Autodesk Fusion 360 part; units mm, degrees
(part 3 of 6)
  spline S37 degree 5 poles (53.0142, 47.6687) (53.0234, 47.6622) (53.0419, 47.6493) (53.0695, 47.6299) (53.1065, 47.6042) (53.1527, 47.5723) (53.1991, 47.5406) (53.2455, 47.5092) (53.292, 47.478) (53.3386, 47.4471) (53.3852, 47.4164) (53.4319, 47.3859) (53.4787, 47.3557) (53.5256, 47.3258) (53.5726, 47.2961) (53.6196, 47.2667) (53.6667, 47.2375) (53.7139, 47.2086) (53.7612, 47.1799) (53.8085, 47.1515) (53.8559, 47.1233) (53.9034, 47.0955) (53.951, 47.0679) (53.9986, 47.0405) (54.0463, 47.0135) (54.0941, 46.9867) (54.142, 46.9602) (54.1899, 46.9339) (54.2379, 46.908) (54.286, 46.8823) (54.3341, 46.8569) (54.3823, 46.8318) (54.4306, 46.807) (54.4789, 46.7825) (54.5273, 46.7583) (54.5758, 46.7344) (54.6244, 46.7108) (54.673, 46.6875) (54.7217, 46.6646) (54.7704, 46.6419) (54.8193, 46.6196) (54.8682, 46.5976) (54.9171, 46.5759) (54.9662, 46.5546) (55.0152, 46.5336) (55.0644, 46.5129) (55.1136, 46.4926) (55.1629, 46.4726) (55.2123, 46.453) (55.2617, 46.4338) (55.3112, 46.4149) (55.3607, 46.3965) (55.4103, 46.3784) (55.46, 46.3608) (55.5098, 46.3436) (55.5596, 46.3268) (55.6095, 46.3104) (55.6594, 46.2943) (55.7094, 46.2787) (55.7594, 46.2635) (55.8095, 46.2488) (55.8597, 46.2348) (55.91, 46.2215) (55.9604, 46.2089) (56.0108, 46.1968) (56.0613, 46.1852) (56.1118, 46.1739) (56.1624, 46.163) (56.213, 46.1525) (56.2636, 46.143) (56.3144, 46.1348) (56.3552, 46.1299) (56.3859, 46.1272) (56.4064, 46.126) (56.4167, 46.1255) knots -1 -1 -1 -1 -1 -1 -0.98571429 -0.97142857 -0.95714286 -0.94285714 -0.92857143 -0.91428571 -0.9 -0.88571429 -0.87142857 -0.85714286 -0.84285714 -0.82857143 -0.81428571 -0.8 -0.78571429 -0.77142857 -0.75714286 -0.74285714 -0.72857143 -0.71428571 -0.7 -0.68571429 -0.67142857 -0.65714286 -0.64285714 -0.62857143 -0.61428571 -0.6 -0.58571429 -0.57142857 -0.55714286 -0.54285714 -0.52857143 -0.51428571 -0.5 -0.48571429 -0.47142857 -0.45714286 -0.44285714 -0.42857143 -0.41428571 -0.4 -0.38571429 -0.37142857 -0.35714286 -0.34285714 -0.32857143 -0.31428571 -0.3 -0.28571429 -0.27142857 -0.25714286 -0.24285714 -0.22857143 -0.21428571 -0.2 -0.18571429 -0.17142857 -0.15714286 -0.14285714 -0.12857143 -0.11428571 -0.1 -0.08571429 -0.07142857 -0.05714286 -0.04285714 -0.02857143 -0.01428571 0 0 0 0 0 0
  line L37 (56.4167, 46.1255) -> (56.9142, 46.1012)
  arc A75 (57.3897, 45.5888) -> (56.9142, 46.1012) centre (56.8899, 45.6018) ccw
  arc A76 (57.3897, 45.5888) -> (57.3897, 44.4112) centre (79.882, 45) ccw
  arc A77 (56.9142, 43.8988) -> (57.3897, 44.4112) centre (56.8899, 44.3982) ccw
  line L38 (56.9142, 43.8988) -> (56.4167, 43.8745)
  spline S38 degree 5 poles (56.4167, 43.8745) (56.4064, 43.874) (56.3859, 43.8728) (56.3552, 43.8701) (56.3144, 43.8652) (56.2636, 43.857) (56.213, 43.8475) (56.1624, 43.837) (56.1118, 43.8261) (56.0613, 43.8148) (56.0108, 43.8032) (55.9604, 43.7911) (55.91, 43.7785) (55.8597, 43.7652) (55.8095, 43.7512) (55.7594, 43.7365) (55.7094, 43.7213) (55.6594, 43.7057) (55.6095, 43.6896) (55.5596, 43.6732) (55.5098, 43.6564) (55.46, 43.6392) (55.4103, 43.6216) (55.3607, 43.6035) (55.3112, 43.5851) (55.2617, 43.5662) (55.2123, 43.547) (55.1629, 43.5274) (55.1136, 43.5074) (55.0644, 43.4871) (55.0152, 43.4664) (54.9662, 43.4454) (54.9171, 43.4241) (54.8682, 43.4024) (54.8193, 43.3804) (54.7704, 43.3581) (54.7217, 43.3354) (54.673, 43.3125) (54.6244, 43.2892) (54.5758, 43.2656) (54.5273, 43.2417) (54.4789, 43.2175) (54.4306, 43.193) (54.3823, 43.1682) (54.3341, 43.1431) (54.286, 43.1177) (54.2379, 43.092) (54.1899, 43.0661) (54.142, 43.0398) (54.0941, 43.0133) (54.0463, 42.9865) (53.9986, 42.9595) (53.951, 42.9321) (53.9034, 42.9045) (53.8559, 42.8767) (53.8085, 42.8485) (53.7612, 42.8201) (53.7139, 42.7914) (53.6667, 42.7625) (53.6196, 42.7333) (53.5726, 42.7039) (53.5256, 42.6742) (53.4787, 42.6443) (53.4319, 42.6141) (53.3852, 42.5836) (53.3386, 42.5529) (53.292, 42.522) (53.2455, 42.4908) (53.1991, 42.4594) (53.1527, 42.4277) (53.1065, 42.3958) (53.0695, 42.3701) (53.0419, 42.3507) (53.0234, 42.3378) (53.0142, 42.3313) knots 0 0 0 0 0 0 0.01428571 0.02857143 0.04285714 0.05714286 0.07142857 0.08571429 0.1 0.11428571 0.12857143 0.14285714 0.15714286 0.17142857 0.18571429 0.2 0.21428571 0.22857143 0.24285714 0.25714286 0.27142857 0.28571429 0.3 0.31428571 0.32857143 0.34285714 0.35714286 0.37142857 0.38571429 0.4 0.41428571 0.42857143 0.44285714 0.45714286 0.47142857 0.48571429 0.5 0.51428571 0.52857143 0.54285714 0.55714286 0.57142857 0.58571429 0.6 0.61428571 0.62857143 0.64285714 0.65714286 0.67142857 0.68571429 0.7 0.71428571 0.72857143 0.74285714 0.75714286 0.77142857 0.78571429 0.8 0.81428571 0.82857143 0.84285714 0.85714286 0.87142857 0.88571429 0.9 0.91428571 0.92857143 0.94285714 0.95714286 0.97142857 0.98571429 1 1 1 1 1 1
  arc A78 (53.0142, 42.3313) -> (53.1946, 40.9031) centre (79.882, 45) ccw
  spline S39 degree 5 poles (53.1946, 40.9031) (53.2052, 40.8991) (53.2263, 40.8912) (53.2579, 40.8793) (53.3001, 40.8635) (53.3528, 40.8441) (53.4055, 40.825) (53.4583, 40.8061) (53.5111, 40.7875) (53.5639, 40.7691) (53.6167, 40.751) (53.6696, 40.7331) (53.7224, 40.7155) (53.7753, 40.6982) (53.8281, 40.6811) (53.881, 40.6643) (53.9339, 40.6477) (53.9868, 40.6314) (54.0397, 40.6154) (54.0926, 40.5997) (54.1455, 40.5842) (54.1985, 40.569) (54.2514, 40.5541) (54.3043, 40.5395) (54.3573, 40.5251) (54.4102, 40.5111) (54.4632, 40.4973) (54.5161, 40.4838) (54.569, 40.4706) (54.622, 40.4577) (54.6749, 40.4451) (54.7279, 40.4328) (54.7808, 40.4207) (54.8337, 40.409) (54.8866, 40.3976) (54.9395, 40.3865) (54.9924, 40.3758) (55.0453, 40.3653) (55.0982, 40.3552) (55.151, 40.3453) (55.2039, 40.3358) (55.2567, 40.3267) (55.3095, 40.3179) (55.3623, 40.3094) (55.4151, 40.3013) (55.4679, 40.2935) (55.5206, 40.2861) (55.5733, 40.279) (55.626, 40.2723) (55.6786, 40.2659) (55.7312, 40.2599) (55.7838, 40.2544) (55.8364, 40.2493) (55.8889, 40.2446) (55.9413, 40.2403) (55.9938, 40.2364) (56.0461, 40.2329) (56.0985, 40.2297) (56.1508, 40.227) (56.2031, 40.2247) (56.2552, 40.223) (56.3073, 40.2219) (56.3594, 40.2215) (56.4113, 40.2218) (56.4632, 40.2227) (56.5149, 40.224) (56.5667, 40.2256) (56.6183, 40.2276) (56.6699, 40.2301) (56.7214, 40.2334) (56.7726, 40.2381) (56.8133, 40.2435) (56.8437, 40.2486) (56.8639, 40.2525) (56.874, 40.2545) knots -1 -1 -1 -1 -1 -1 -0.98571429 -0.97142857 -0.95714286 -0.94285714 -0.92857143 -0.91428571 -0.9 -0.88571429 -0.87142857 -0.85714286 -0.84285714 -0.82857143 -0.81428571 -0.8 -0.78571429 -0.77142857 -0.75714286 -0.74285714 -0.72857143 -0.71428571 -0.7 -0.68571429 -0.67142857 -0.65714286 -0.64285714 -0.62857143 -0.61428571 -0.6 -0.58571429 -0.57142857 -0.55714286 -0.54285714 -0.52857143 -0.51428571 -0.5 -0.48571429 -0.47142857 -0.45714286 -0.44285714 -0.42857143 -0.41428571 -0.4 -0.38571429 -0.37142857 -0.35714286 -0.34285714 -0.32857143 -0.31428571 -0.3 -0.28571429 -0.27142857 -0.25714286 -0.24285714 -0.22857143 -0.21428571 -0.2 -0.18571429 -0.17142857 -0.15714286 -0.14285714 -0.12857143 -0.11428571 -0.1 -0.08571429 -0.07142857 -0.05714286 -0.04285714 -0.02857143 -0.01428571 0 0 0 0 0 0
  line L39 (56.874, 40.2545) -> (57.3619, 40.3548)
  arc A79 (57.9499, 39.9767) -> (57.3619, 40.3548) centre (57.4626, 39.865) ccw
  arc A80 (57.9499, 39.9767) -> (58.2428, 38.8361) centre (79.882, 45) ccw
  arc A81 (57.9097, 38.2215) -> (58.2428, 38.8361) centre (57.7619, 38.6992) ccw
  line L40 (57.9097, 38.2215) -> (57.4338, 38.0743)
  spline S40 degree 5 poles (57.4338, 38.0743) (57.424, 38.0712) (57.4044, 38.0649) (57.3753, 38.0547) (57.337, 38.0398) (57.2899, 38.0193) (57.2432, 37.9974) (57.1968, 37.9747) (57.1506, 37.9515) (57.1044, 37.9281) (57.0584, 37.9043) (57.0126, 37.88) (56.9669, 37.8553) (56.9215, 37.8299) (56.8764, 37.8038) (56.8315, 37.7772) (56.7868, 37.75) (56.7423, 37.7224) (56.6979, 37.6944) (56.6537, 37.6661) (56.6096, 37.6375) (56.5657, 37.6084) (56.522, 37.579) (56.4784, 37.5492) (56.435, 37.519) (56.3917, 37.4884) (56.3487, 37.4575) (56.3057, 37.4262) (56.263, 37.3946) (56.2203, 37.3627) (56.1779, 37.3305) (56.1355, 37.298) (56.0934, 37.2651) (56.0513, 37.2319) (56.0094, 37.1985) (55.9677, 37.1647) (55.9261, 37.1306) (55.8847, 37.0962) (55.8434, 37.0616) (55.8022, 37.0267) (55.7612, 36.9915) (55.7203, 36.956) (55.6796, 36.9202) (55.639, 36.8842) (55.5985, 36.8479) (55.5582, 36.8114) (55.518, 36.7745) (55.478, 36.7375) (55.4381, 36.7001) (55.3984, 36.6626) (55.3587, 36.6247) (55.3193, 36.5866) (55.2799, 36.5483) (55.2407, 36.5097) (55.2017, 36.4709) (55.1627, 36.4319) (55.1239, 36.3926) (55.0853, 36.3531) (55.0468, 36.3133) (55.0084, 36.2734) (54.9702, 36.2331) (54.9321, 36.1927) (54.8941, 36.152) (54.8563, 36.1112) (54.8186, 36.07) (54.781, 36.0287) (54.7436, 35.9872) (54.7063, 35.9454) (54.6692, 35.9034) (54.6322, 35.8613) (54.5953, 35.8189) (54.5659, 35.7848) (54.544, 35.7591) (54.5293, 35.7419) (54.522, 35.7334) knots 0 0 0 0 0 0 0.01428571 0.02857143 0.04285714 0.05714286 0.07142857 0.08571429 0.1 0.11428571 0.12857143 0.14285714 0.15714286 0.17142857 0.18571429 0.2 0.21428571 0.22857143 0.24285714 0.25714286 0.27142857 0.28571429 0.3 0.31428571 0.32857143 0.34285714 0.35714286 0.37142857 0.38571429 0.4 0.41428571 0.42857143 0.44285714 0.45714286 0.47142857 0.48571429 0.5 0.51428571 0.52857143 0.54285714 0.55714286 0.57142857 0.58571429 0.6 0.61428571 0.62857143 0.64285714 0.65714286 0.67142857 0.68571429 0.7 0.71428571 0.72857143 0.74285714 0.75714286 0.77142857 0.78571429 0.8 0.81428571 0.82857143 0.84285714 0.85714286 0.87142857 0.88571429 0.9 0.91428571 0.92857143 0.94285714 0.95714286 0.97142857 0.98571429 1 1 1 1 1 1
  arc A82 (54.522, 35.7334) -> (55.0519, 34.395) centre (79.882, 45) ccw
  spline S41 degree 5 poles (55.0519, 34.395) (55.0631, 34.3937) (55.0855, 34.3912) (55.1191, 34.3876) (55.1639, 34.3828) (55.2198, 34.3772) (55.2756, 34.3717) (55.3314, 34.3666) (55.3872, 34.3616) (55.4429, 34.357) (55.4986, 34.3526) (55.5542, 34.3484) (55.6098, 34.3445) (55.6653, 34.3408) (55.7207, 34.3374) (55.7761, 34.3343) (55.8315, 34.3314) (55.8868, 34.3288) (55.942, 34.3265) (55.9972, 34.3244) (56.0523, 34.3225) (56.1073, 34.321) (56.1623, 34.3197) (56.2172, 34.3187) (56.272, 34.318) (56.3268, 34.3175) (56.3815, 34.3173) (56.4362, 34.3174) (56.4907, 34.3178) (56.5452, 34.3185) (56.5996, 34.3194) (56.654, 34.3207) (56.7082, 34.3222) (56.7624, 34.324) (56.8165, 34.3261) (56.8705, 34.3285) (56.9244, 34.3313) (56.9782, 34.3343) (57.0319, 34.3376) (57.0856, 34.3412) (57.1391, 34.3452) (57.1926, 34.3494) (57.2459, 34.354) (57.2992, 34.359) (57.3523, 34.3642) (57.4053, 34.3698) (57.4582, 34.3757) (57.5111, 34.382) (57.5638, 34.3886) (57.6163, 34.3955) (57.6688, 34.4028) (57.7211, 34.4105) (57.7733, 34.4186) (57.8253, 34.4271) (57.8772, 34.436) (57.9289, 34.4453) (57.9805, 34.4549) (58.032, 34.4649) (58.0834, 34.4752) (58.1345, 34.486) (58.1855, 34.4974) (58.2362, 34.5093) (58.2867, 34.5218) (58.337, 34.535) (58.387, 34.5487) (58.4368, 34.5629) (58.4865, 34.5773) (58.5361, 34.5921) (58.5854, 34.6073) (58.6344, 34.6233) (58.6829, 34.6407) (58.721, 34.656) (58.7491, 34.6685) (58.7677, 34.6773) (58.777, 34.6818) knots -1 -1 -1 -1 -1 -1 -0.98571429 -0.97142857 -0.95714286 -0.94285714 -0.92857143 -0.91428571 -0.9 -0.88571429 -0.87142857 -0.85714286 -0.84285714 -0.82857143 -0.81428571 -0.8 -0.78571429 -0.77142857 -0.75714286 -0.74285714 -0.72857143 -0.71428571 -0.7 -0.68571429 -0.67142857 -0.65714286 -0.64285714 -0.62857143 -0.61428571 -0.6 -0.58571429 -0.57142857 -0.55714286 -0.54285714 -0.52857143 -0.51428571 -0.5 -0.48571429 -0.47142857 -0.45714286 -0.44285714 -0.42857143 -0.41428571 -0.4 -0.38571429 -0.37142857 -0.35714286 -0.34285714 -0.32857143 -0.31428571 -0.3 -0.28571429 -0.27142857 -0.25714286 -0.24285714 -0.22857143 -0.21428571 -0.2 -0.18571429 -0.17142857 -0.15714286 -0.14285714 -0.12857143 -0.11428571 -0.1 -0.08571429 -0.07142857 -0.05714286 -0.04285714 -0.02857143 -0.01428571 0 0 0 0 0 0
  line L41 (58.777, 34.6818) -> (59.2247, 34.9002)
  arc A83 (59.8882, 34.6802) -> (59.2247, 34.9002) centre (59.4439, 34.4509) ccw
  arc A84 (59.8882, 34.6802) -> (60.4555, 33.6483) centre (79.882, 45) ccw
  arc A85 (60.2857, 32.9702) -> (60.4555, 33.6483) centre (60.0238, 33.3961) ccw
  line L42 (60.2857, 32.9702) -> (59.8614, 32.7092)
  spline S42 degree 5 poles (59.8614, 32.7092) (59.8526, 32.7038) (59.8353, 32.6928) (59.8096, 32.6757) (59.7763, 32.6518) (59.7357, 32.6202) (59.6959, 32.5874) (59.6566, 32.5538) (59.6176, 32.5199) (59.5788, 32.4857) (59.5401, 32.4512) (59.5017, 32.4163) (59.4637, 32.381) (59.426, 32.3451) (59.3888, 32.3086) (59.3519, 32.2717) (59.3154, 32.2342) (59.2791, 32.1964) (59.2431, 32.1583) (59.2073, 32.1199) (59.1718, 32.0812) (59.1364, 32.0421) (59.1014, 32.0028) (59.0666, 31.9631) (59.0321, 31.923) (58.9978, 31.8826) (58.9638, 31.842) (58.93, 31.801) (58.8964, 31.7598) (58.863, 31.7182) (58.8299, 31.6765) (58.797, 31.6344) (58.7643, 31.5921) (58.7318, 31.5495) (58.6996, 31.5067) (58.6676, 31.4636) (58.6358, 31.4202) (58.6042, 31.3767) (58.5728, 31.3328) (58.5416, 31.2888) (58.5106, 31.2445) (58.4799, 31.1999) (58.4493, 31.1552) (58.4189, 31.1102) (58.3888, 31.065) (58.3588, 31.0195) (58.3291, 30.9739) (58.2995, 30.928) (58.2702, 30.8819) (58.241, 30.8356) (58.212, 30.7892) (58.1833, 30.7425) (58.1547, 30.6955) (58.1263, 30.6484) (58.0981, 30.6011) (58.0701, 30.5536) (58.0423, 30.5059) (58.0147, 30.4581) (57.9873, 30.41) (57.9601, 30.3617) (57.933, 30.3132) (57.9062, 30.2646) (57.8795, 30.2158) (57.8531, 30.1668) (57.8268, 30.1176) (57.8007, 30.0682) (57.7748, 30.0187) (57.7491, 29.9689) (57.7235, 29.9191) (57.6982, 29.869) (57.673, 29.8187) (57.653, 29.7784) (57.6381, 29.7481) (57.6282, 29.7278) (57.6233, 29.7177) knots 0 0 0 0 0 0 0.01428571 0.02857143 0.04285714 0.05714286 0.07142857 0.08571429 0.1 0.11428571 0.12857143 0.14285714 0.15714286 0.17142857 0.18571429 0.2 0.21428571 0.22857143 0.24285714 0.25714286 0.27142857 0.28571429 0.3 0.31428571 0.32857143 0.34285714 0.35714286 0.37142857 0.38571429 0.4 0.41428571 0.42857143 0.44285714 0.45714286 0.47142857 0.48571429 0.5 0.51428571 0.52857143 0.54285714 0.55714286 0.57142857 0.58571429 0.6 0.61428571 0.62857143 0.64285714 0.65714286 0.67142857 0.68571429 0.7 0.71428571 0.72857143 0.74285714 0.75714286 0.77142857 0.78571429 0.8 0.81428571 0.82857143 0.84285714 0.85714286 0.87142857 0.88571429 0.9 0.91428571 0.92857143 0.94285714 0.95714286 0.97142857 0.98571429 1 1 1 1 1 1
  arc A86 (57.6233, 29.7177) -> (58.4694, 28.5532) centre (79.882, 45) ccw
  spline S43 degree 5 poles (58.4694, 28.5532) (58.4805, 28.5547) (58.5028, 28.5579) (58.5363, 28.5627) (58.5808, 28.5692) (58.6364, 28.5776) (58.6918, 28.5863) (58.7472, 28.5952) (58.8024, 28.6043) (58.8575, 28.6136) (58.9125, 28.6231) (58.9675, 28.6329) (59.0222, 28.643) (59.0769, 28.6532) (59.1315, 28.6637) (59.1859, 28.6745) (59.2402, 28.6855) (59.2944, 28.6967) (59.3485, 28.7081) (59.4025, 28.7198) (59.4563, 28.7318) (59.51, 28.744) (59.5636, 28.7564) (59.617, 28.7691) (59.6703, 28.782) (59.7235, 28.7952) (59.7765, 28.8086) (59.8294, 28.8223) (59.8822, 28.8362) (59.9348, 28.8504) (59.9872, 28.8649) (60.0395, 28.8796) (60.0917, 28.8946) (60.1437, 28.9098) (60.1956, 28.9253) (60.2473, 28.9411) (60.2988, 28.9571) (60.3502, 28.9734) (60.4015, 28.99) (60.4525, 29.0069) (60.5034, 29.024) (60.5541, 29.0414) (60.6046, 29.0591) (60.655, 29.0771) (60.7051, 29.0955) (60.7551, 29.1141) (60.8049, 29.1329) (60.8545, 29.1521) (60.9039, 29.1716) (60.9531, 29.1914) (61.0021, 29.2115) (61.0508, 29.232) (61.0993, 29.2528) (61.1476, 29.274) (61.1957, 29.2955) (61.2435, 29.3174) (61.2911, 29.3395) (61.3384, 29.362) (61.3856, 29.3848) (61.4325, 29.408) (61.479, 29.4316) (61.5252, 29.4558) (61.571, 29.4805) (61.6164, 29.5057) (61.6614, 29.5315) (61.7061, 29.5576) (61.7507, 29.5839) (61.795, 29.6106) (61.839, 29.6376) (61.8825, 29.6653) (61.9251, 29.6941) (61.9582, 29.7184) (61.9824, 29.7375) (61.9982, 29.7507) (62.0061, 29.7573) knots -1 -1 -1 -1 -1 -1 -0.98571429 -0.97142857 -0.95714286 -0.94285714 -0.92857143 -0.91428571 -0.9 -0.88571429 -0.87142857 -0.85714286 -0.84285714 -0.82857143 -0.81428571 -0.8 -0.78571429 -0.77142857 -0.75714286 -0.74285714 -0.72857143 -0.71428571 -0.7 -0.68571429 -0.67142857 -0.65714286 -0.64285714 -0.62857143 -0.61428571 -0.6 -0.58571429 -0.57142857 -0.55714286 -0.54285714 -0.52857143 -0.51428571 -0.5 -0.48571429 -0.47142857 -0.45714286 -0.44285714 -0.42857143 -0.41428571 -0.4 -0.38571429 -0.37142857 -0.35714286 -0.34285714 -0.32857143 -0.31428571 -0.3 -0.28571429 -0.27142857 -0.25714286 -0.24285714 -0.22857143 -0.21428571 -0.2 -0.18571429 -0.17142857 -0.15714286 -0.14285714 -0.12857143 -0.11428571 -0.1 -0.08571429 -0.07142857 -0.05714286 -0.04285714 -0.02857143 -0.01428571 0 0 0 0 0 0
  line L43 (62.0061, 29.7573) -> (62.3854, 30.0802)
  arc A87 (63.0828, 30.0321) -> (62.3854, 30.0802) centre (62.7095, 29.6995) ccw
  arc A88 (63.0828, 30.0321) -> (63.8889, 29.1738) centre (79.882, 45) ccw
  arc A89 (63.8931, 28.4747) -> (63.8889, 29.1738) centre (63.5335, 28.8221) ccw
  line L44 (63.8931, 28.4747) -> (63.547, 28.1164)
  spline S44 degree 5 poles (63.547, 28.1164) (63.5398, 28.109) (63.5257, 28.0941) (63.5052, 28.0711) (63.4788, 28.0396) (63.4473, 27.9989) (63.417, 27.9573) (63.3873, 27.915) (63.3579, 27.8724) (63.3288, 27.8296) (63.2999, 27.7866) (63.2714, 27.7433) (63.2434, 27.6996) (63.2158, 27.6555) (63.1888, 27.6109) (63.1623, 27.5659) (63.1362, 27.5206) (63.1105, 27.4749) (63.0851, 27.4291) (63.06, 27.3829) (63.0352, 27.3366) (63.0107, 27.29) (62.9865, 27.2432) (62.9627, 27.196) (62.9392, 27.1487) (62.9161, 27.101) (62.8932, 27.0532) (62.8707, 27.0051) (62.8484, 26.9568) (62.8264, 26.9083) (62.8047, 26.8596) (62.7833, 26.8107) (62.7622, 26.7616) (62.7413, 26.7123) (62.7207, 26.6628) (62.7004, 26.613) (62.6804, 26.5632) (62.6606, 26.5131) (62.6411, 26.4628) (62.6219, 26.4124) (62.6029, 26.3618) (62.5842, 26.311) (62.5657, 26.26) (62.5475, 26.2089) (62.5295, 26.1576) (62.5118, 26.1062) (62.4943, 26.0545) (62.4771, 26.0028) (62.4601, 25.9508) (62.4434, 25.8987) (62.4269, 25.8465) (62.4107, 25.7941) (62.3947, 25.7416) (62.3789, 25.6889) (62.3634, 25.6361) (62.3481, 25.5831) (62.333, 25.53) (62.3182, 25.4767) (62.3036, 25.4234) (62.2892, 25.3698) (62.2751, 25.3162) (62.2612, 25.2624) (62.2475, 25.2085) (62.234, 25.1544) (62.2208, 25.1002) (62.2078, 25.0459) (62.195, 24.9915) (62.1825, 24.9369) (62.1701, 24.8823) (62.158, 24.8275) (62.1462, 24.7725) (62.1368, 24.7285) (62.1299, 24.6954) (62.1254, 24.6734) (62.1231, 24.6623) knots 0 0 0 0 0 0 0.01428571 0.02857143 0.04285714 0.05714286 0.07142857 0.08571429 0.1 0.11428571 0.12857143 0.14285714 0.15714286 0.17142857 0.18571429 0.2 0.21428571 0.22857143 0.24285714 0.25714286 0.27142857 0.28571429 0.3 0.31428571 0.32857143 0.34285714 0.35714286 0.37142857 0.38571429 0.4 0.41428571 0.42857143 0.44285714 0.45714286 0.47142857 0.48571429 0.5 0.51428571 0.52857143 0.54285714 0.55714286 0.57142857 0.58571429 0.6 0.61428571 0.62857143 0.64285714 0.65714286 0.67142857 0.68571429 0.7 0.71428571 0.72857143 0.74285714 0.75714286 0.77142857 0.78571429 0.8 0.81428571 0.82857143 0.84285714 0.85714286 0.87142857 0.88571429 0.9 0.91428571 0.92857143 0.94285714 0.95714286 0.97142857 0.98571429 1 1 1 1 1 1
  arc A90 (62.1231, 24.6623) -> (63.2322, 23.7448) centre (79.882, 45) ccw
  spline S45 degree 5 poles (63.2322, 23.7448) (63.2427, 23.7491) (63.2635, 23.7577) (63.2947, 23.7706) (63.3362, 23.788) (63.3879, 23.81) (63.4395, 23.8322) (63.4909, 23.8545) (63.5421, 23.8771) (63.5932, 23.8998) (63.6441, 23.9228) (63.6948, 23.9459) (63.7454, 23.9692) (63.7958, 23.9928) (63.8461, 24.0165) (63.8961, 24.0405) (63.946, 24.0646) (63.9957, 24.089) (64.0452, 24.1135) (64.0946, 24.1383) (64.1437, 24.1632) (64.1927, 24.1884) (64.2415, 24.2137) (64.2901, 24.2393) (64.3385, 24.2651) (64.3868, 24.2911) (64.4348, 24.3173) (64.4826, 24.3437) (64.5303, 24.3703) (64.5777, 24.3971) (64.6249, 24.4242) (64.6719, 24.4514) (64.7187, 24.4789) (64.7653, 24.5066) (64.8117, 24.5345) (64.8579, 24.5626) (64.9038, 24.591) (64.9495, 24.6196) (64.995, 24.6484) (65.0403, 24.6774) (65.0853, 24.7066) (65.1301, 24.7361) (65.1746, 24.7659) (65.2189, 24.7958) (65.2629, 24.826) (65.3067, 24.8565) (65.3502, 24.8871) (65.3935, 24.9181) (65.4365, 24.9492) (65.4792, 24.9806) (65.5216, 25.0123) (65.5638, 25.0442) (65.6056, 25.0765) (65.6471, 25.109) (65.6883, 25.1418) (65.7291, 25.1748) (65.7697, 25.2081) (65.81, 25.2417) (65.85, 25.2755) (65.8897, 25.3096) (65.9289, 25.3441) (65.9676, 25.379) (66.0058, 25.4143) (66.0435, 25.45) (66.0807, 25.4862) (66.1175, 25.5226) (66.1541, 25.5592) (66.1905, 25.596) (66.2264, 25.6331) (66.2616, 25.6707) (66.2957, 25.7093) (66.3217, 25.7411) (66.3404, 25.7656) (66.3524, 25.7822) (66.3584, 25.7906) knots -1 -1 -1 -1 -1 -1 -0.98571429 -0.97142857 -0.95714286 -0.94285714 -0.92857143 -0.91428571 -0.9 -0.88571429 -0.87142857 -0.85714286 -0.84285714 -0.82857143 -0.81428571 -0.8 -0.78571429 -0.77142857 -0.75714286 -0.74285714 -0.72857143 -0.71428571 -0.7 -0.68571429 -0.67142857 -0.65714286 -0.64285714 -0.62857143 -0.61428571 -0.6 -0.58571429 -0.57142857 -0.55714286 -0.54285714 -0.52857143 -0.51428571 -0.5 -0.48571429 -0.47142857 -0.45714286 -0.44285714 -0.42857143 -0.41428571 -0.4 -0.38571429 -0.37142857 -0.35714286 -0.34285714 -0.32857143 -0.31428571 -0.3 -0.28571429 -0.27142857 -0.25714286 -0.24285714 -0.22857143 -0.21428571 -0.2 -0.18571429 -0.17142857 -0.15714286 -0.14285714 -0.12857143 -0.11428571 -0.1 -0.08571429 -0.07142857 -0.05714286 -0.04285714 -0.02857143 -0.01428571 0 0 0 0 0 0
  line L45 (66.3584, 25.7906) -> (66.6454, 26.1977)
  arc A91 (67.3329, 26.3246) -> (66.6454, 26.1977) centre (67.0541, 25.9096) ccw
  arc A92 (67.3329, 26.3246) -> (68.3271, 25.6937) centre (79.882, 45) ccw
  arc A93 (68.5051, 25.0176) -> (68.3271, 25.6937) centre (68.0704, 25.2646) ccw
  line L46 (68.5051, 25.0176) -> (68.2589, 24.5845)
  spline S46 degree 5 poles (68.2589, 24.5845) (68.2539, 24.5755) (68.2439, 24.5576) (68.2297, 24.5302) (68.212, 24.4931) (68.1917, 24.4459) (68.1726, 24.398) (68.1543, 24.3497) (68.1365, 24.3011) (68.1189, 24.2525) (68.1017, 24.2036) (68.0848, 24.1546) (68.0685, 24.1053) (68.0528, 24.0557) (68.0378, 24.0058) (68.0233, 23.9556) (68.0093, 23.9052) (67.9957, 23.8546) (67.9825, 23.8039) (67.9697, 23.753) (67.9572, 23.7019) (67.945, 23.6507) (67.9333, 23.5993) (67.9219, 23.5477) (67.9109, 23.496) (67.9004, 23.4441) (67.8901, 23.3921) (67.8803, 23.3399) (67.8707, 23.2876) (67.8615, 23.2351) (67.8526, 23.1826) (67.844, 23.1299) (67.8357, 23.077) (67.8278, 23.0241) (67.8202, 22.971) (67.8129, 22.9178) (67.8059, 22.8645) (67.7992, 22.8111) (67.7928, 22.7576) (67.7867, 22.7039) (67.7809, 22.6502) (67.7754, 22.5963) (67.7702, 22.5424) (67.7652, 22.4883) (67.7606, 22.4342) (67.7562, 22.3799) (67.7522, 22.3256) (67.7484, 22.2712) (67.7448, 22.2167) (67.7416, 22.162) (67.7386, 22.1073) (67.7359, 22.0526) (67.7334, 21.9977) (67.7313, 21.9427) (67.7294, 21.8877) (67.7277, 21.8326) (67.7263, 21.7774) (67.7252, 21.7221) (67.7243, 21.6668) (67.7237, 21.6114) (67.7234, 21.5559) (67.7233, 21.5003) (67.7235, 21.4447) (67.7239, 21.389) (67.7245, 21.3332) (67.7254, 21.2774) (67.7266, 21.2215) (67.728, 21.1656) (67.7297, 21.1095) (67.7316, 21.0534) (67.7337, 20.9973) (67.7356, 20.9523) (67.7372, 20.9186) (67.7383, 20.8961) (67.7388, 20.8848) knots 0 0 0 0 0 0 0.01428571 0.02857143 0.04285714 0.05714286 0.07142857 0.08571429 0.1 0.11428571 0.12857143 0.14285714 0.15714286 0.17142857 0.18571429 0.2 0.21428571 0.22857143 0.24285714 0.25714286 0.27142857 0.28571429 0.3 0.31428571 0.32857143 0.34285714 0.35714286 0.37142857 0.38571429 0.4 0.41428571 0.42857143 0.44285714 0.45714286 0.47142857 0.48571429 0.5 0.51428571 0.52857143 0.54285714 0.55714286 0.57142857 0.58571429 0.6 0.61428571 0.62857143 0.64285714 0.65714286 0.67142857 0.68571429 0.7 0.71428571 0.72857143 0.74285714 0.75714286 0.77142857 0.78571429 0.8 0.81428571 0.82857143 0.84285714 0.85714286 0.87142857 0.88571429 0.9 0.91428571 0.92857143 0.94285714 0.95714286 0.97142857 0.98571429 1 1 1 1 1 1
  arc A94 (67.7388, 20.8848) -> (69.0413, 20.2719) centre (79.882, 45) ccw
  spline S47 degree 5 poles (69.0413, 20.2719) (69.0503, 20.2787) (69.0684, 20.2922) (69.0954, 20.3125) (69.1312, 20.3397) (69.1759, 20.3738) (69.2203, 20.4081) (69.2645, 20.4425) (69.3085, 20.4771) (69.3523, 20.5119) (69.3959, 20.5467) (69.4393, 20.5818) (69.4825, 20.617) (69.5255, 20.6523) (69.5682, 20.6878) (69.6108, 20.7234) (69.6531, 20.7592) (69.6952, 20.7952) (69.737, 20.8312) (69.7787, 20.8675) (69.8201, 20.9039) (69.8613, 20.9404) (69.9022, 20.9771) (69.943, 21.014) (69.9834, 21.051) (70.0237, 21.0882) (70.0637, 21.1255) (70.1034, 21.163) (70.143, 21.2006) (70.1822, 21.2384) (70.2212, 21.2763) (70.26, 21.3144) (70.2985, 21.3526) (70.3367, 21.3911) (70.3747, 21.4296) (70.4124, 21.4683) (70.4499, 21.5072) (70.487, 21.5463) (70.5239, 21.5855) (70.5606, 21.6249) (70.5969, 21.6644) (70.6329, 21.7041) (70.6687, 21.744) (70.7041, 21.784) (70.7392, 21.8242) (70.7741, 21.8646) (70.8086, 21.9051) (70.8428, 21.9458) (70.8767, 21.9867) (70.9103, 22.0277) (70.9435, 22.069) (70.9764, 22.1104) (71.0089, 22.152) (71.041, 22.1938) (71.0727, 22.2358) (71.1041, 22.278) (71.1351, 22.3204) (71.1658, 22.3629) (71.1962, 22.4056) (71.2261, 22.4485) (71.2555, 22.4916) (71.2843, 22.535) (71.3125, 22.5787) (71.3401, 22.6227) (71.3672, 22.667) (71.3938, 22.7114) (71.4202, 22.756) (71.4462, 22.8007) (71.4718, 22.8455) (71.4965, 22.8908) (71.5199, 22.9365) (71.5372, 22.9738) (71.5492, 23.0022) (71.5568, 23.0213) (71.5604, 23.0309) knots -1 -1 -1 -1 -1 -1 -0.98571429 -0.97142857 -0.95714286 -0.94285714 -0.92857143 -0.91428571 -0.9 -0.88571429 -0.87142857 -0.85714286 -0.84285714 -0.82857143 -0.81428571 -0.8 -0.78571429 -0.77142857 -0.75714286 -0.74285714 -0.72857143 -0.71428571 -0.7 -0.68571429 -0.67142857 -0.65714286 -0.64285714 -0.62857143 -0.61428571 -0.6 -0.58571429 -0.57142857 -0.55714286 -0.54285714 -0.52857143 -0.51428571 -0.5 -0.48571429 -0.47142857 -0.45714286 -0.44285714 -0.42857143 -0.41428571 -0.4 -0.38571429 -0.37142857 -0.35714286 -0.34285714 -0.32857143 -0.31428571 -0.3 -0.28571429 -0.27142857 -0.25714286 -0.24285714 -0.22857143 -0.21428571 -0.2 -0.18571429 -0.17142857 -0.15714286 -0.14285714 -0.12857143 -0.11428571 -0.1 -0.08571429 -0.07142857 -0.05714286 -0.04285714 -0.02857143 -0.01428571 0 0 0 0 0 0
  line L47 (71.5604, 23.0309) -> (71.7372, 23.4966)
  arc A95 (72.3716, 23.7905) -> (71.7372, 23.4966) centre (72.2047, 23.3192) ccw
  arc A96 (72.3716, 23.7905) -> (73.4915, 23.4266) centre (79.882, 45) ccw
  arc A97 (73.8319, 22.816) -> (73.4915, 23.4266) centre (73.3494, 22.9472) ccw
  line L48 (73.8319, 22.816) -> (73.7012, 22.3353)
  spline S48 degree 5 poles (73.7012, 22.3353) (73.6985, 22.3254) (73.6934, 22.3055) (73.6864, 22.2755) (73.6785, 22.2352) (73.6705, 22.1844) (73.664, 22.1332) (73.6583, 22.0819) (73.6531, 22.0304) (73.6482, 21.9789) (73.6436, 21.9273) (73.6395, 21.8756) (73.636, 21.8238) (73.6331, 21.7719) (73.6309, 21.7198) (73.6294, 21.6676) (73.6283, 21.6153) (73.6278, 21.5629) (73.6276, 21.5105) (73.6278, 21.458) (73.6284, 21.4054) (73.6294, 21.3528) (73.6308, 21.3001) (73.6326, 21.2473) (73.6349, 21.1945) (73.6375, 21.1416) (73.6406, 21.0887) (73.644, 21.0357) (73.6477, 20.9826) (73.6518, 20.9295) (73.6563, 20.8764) (73.6611, 20.8232) (73.6662, 20.77) (73.6717, 20.7167) (73.6775, 20.6634) (73.6837, 20.6101) (73.6901, 20.5567) (73.697, 20.5033) (73.7041, 20.4499) (73.7115, 20.3964) (73.7193, 20.3429) (73.7273, 20.2894) (73.7357, 20.2358) (73.7443, 20.1823) (73.7533, 20.1287) (73.7626, 20.075) (73.7721, 20.0214) (73.782, 19.9677) (73.7921, 19.914) (73.8026, 19.8603) (73.8133, 19.8066) (73.8243, 19.7529) (73.8355, 19.6991) (73.8471, 19.6454) (73.8589, 19.5916) (73.8711, 19.5378) (73.8834, 19.484) (73.8961, 19.4302) (73.909, 19.3764) (73.9222, 19.3225) (73.9357, 19.2687) (73.9494, 19.2149) (73.9634, 19.161) (73.9776, 19.1072) (73.9922, 19.0533) (74.0069, 18.9995) (74.022, 18.9456) (74.0372, 18.8918) (74.0528, 18.8379) (74.0686, 18.7841) (74.0846, 18.7302) (74.0977, 18.6871) (74.1076, 18.6548) (74.1142, 18.6333) (74.1175, 18.6225) knots 0 0 0 0 0 0 0.01428571 0.02857143 0.04285714 0.05714286 0.07142857 0.08571429 0.1 0.11428571 0.12857143 0.14285714 0.15714286 0.17142857 0.18571429 0.2 0.21428571 0.22857143 0.24285714 0.25714286 0.27142857 0.28571429 0.3 0.31428571 0.32857143 0.34285714 0.35714286 0.37142857 0.38571429 0.4 0.41428571 0.42857143 0.44285714 0.45714286 0.47142857 0.48571429 0.5 0.51428571 0.52857143 0.54285714 0.55714286 0.57142857 0.58571429 0.6 0.61428571 0.62857143 0.64285714 0.65714286 0.67142857 0.68571429 0.7 0.71428571 0.72857143 0.74285714 0.75714286 0.77142857 0.78571429 0.8 0.81428571 0.82857143 0.84285714 0.85714286 0.87142857 0.88571429 0.9 0.91428571 0.92857143 0.94285714 0.95714286 0.97142857 0.98571429 1 1 1 1 1 1
  arc A98 (74.1175, 18.6225) -> (75.5315, 18.3528) centre (79.882, 45) ccw
  spline S49 degree 5 poles (75.5315, 18.3528) (75.5386, 18.3616) (75.5527, 18.3792) (75.5738, 18.4056) (75.6017, 18.4408) (75.6365, 18.485) (75.671, 18.5292) (75.7053, 18.5736) (75.7393, 18.618) (75.7731, 18.6626) (75.8067, 18.7072) (75.84, 18.7519) (75.8731, 18.7967) (75.9059, 18.8417) (75.9385, 18.8867) (75.9708, 18.9318) (76.0029, 18.9769) (76.0347, 19.0222) (76.0663, 19.0676) (76.0976, 19.1131) (76.1287, 19.1586) (76.1595, 19.2043) (76.19, 19.25) (76.2203, 19.2958) (76.2503, 19.3417) (76.28, 19.3877) (76.3095, 19.4338) (76.3387, 19.48) (76.3676, 19.5263) (76.3962, 19.5726) (76.4246, 19.6191) (76.4527, 19.6656) (76.4804, 19.7122) (76.5079, 19.759) (76.5351, 19.8058) (76.562, 19.8526) (76.5886, 19.8996) (76.6149, 19.9467) (76.6409, 19.9938) (76.6666, 20.0411) (76.6919, 20.0884) (76.717, 20.1358) (76.7417, 20.1833) (76.766, 20.2309) (76.7901, 20.2786) (76.8138, 20.3264) (76.8371, 20.3742) (76.8602, 20.4221) (76.8828, 20.4702) (76.9051, 20.5183) (76.9271, 20.5665) (76.9486, 20.6148) (76.9697, 20.6632) (76.9904, 20.7116) (77.0107, 20.7602) (77.0306, 20.8089) (77.0501, 20.8576) (77.0693, 20.9064) (77.0881, 20.9553) (77.1064, 21.0043) (77.1241, 21.0534) (77.1413, 21.1027) (77.1577, 21.152) (77.1735, 21.2015) (77.1887, 21.2511) (77.2034, 21.3007) (77.2179, 21.3504) (77.232, 21.4002) (77.2456, 21.45) (77.2583, 21.5) (77.2696, 21.5501) (77.2771, 21.5905) (77.2817, 21.621) (77.2842, 21.6414) (77.2853, 21.6516) knots -1 -1 -1 -1 -1 -1 -0.98571429 -0.97142857 -0.95714286 -0.94285714 -0.92857143 -0.91428571 -0.9 -0.88571429 -0.87142857 -0.85714286 -0.84285714 -0.82857143 -0.81428571 -0.8 -0.78571429 -0.77142857 -0.75714286 -0.74285714 -0.72857143 -0.71428571 -0.7 -0.68571429 -0.67142857 -0.65714286 -0.64285714 -0.62857143 -0.61428571 -0.6 -0.58571429 -0.57142857 -0.55714286 -0.54285714 -0.52857143 -0.51428571 -0.5 -0.48571429 -0.47142857 -0.45714286 -0.44285714 -0.42857143 -0.41428571 -0.4 -0.38571429 -0.37142857 -0.35714286 -0.34285714 -0.32857143 -0.31428571 -0.3 -0.28571429 -0.27142857 -0.25714286 -0.24285714 -0.22857143 -0.21428571 -0.2 -0.18571429 -0.17142857 -0.15714286 -0.14285714 -0.12857143 -0.11428571 -0.1 -0.08571429 -0.07142857 -0.05714286 -0.04285714 -0.02857143 -0.01428571 0 0 0 0 0 0
  line L49 (77.2853, 21.6516) -> (77.3408, 22.1467)
  arc A99 (77.8821, 22.5891) -> (77.3408, 22.1467) centre (77.8377, 22.091) ccw
  line L50 (79.882, 45) -> (99.5642, 63.4828) construction
  line L51 (94.2241, 62.3365) -> (103.1265, 70.6965)
  line L52 (106.9873, 66.5851) -> (98.0849, 58.2252)
  circle A100 centre (110.7338, 73.9718) radius 1.75
  arc A101 (111.7668, 69.0797) -> (105.9162, 75.3099) centre (110.7338, 73.9718) ccw
  arc A102 (103.1265, 70.6965) -> (105.9162, 75.3099) centre (96.281, 77.9862) ccw
  arc A103 (111.7668, 69.0797) -> (106.9873, 66.5851) centre (113.8328, 59.2954) ccw
  circle A104 centre (79.882, 45) radius 0.5
  circle A105 centre (79.882, 45) radius 1.75
  dimension "d193" = 3.5
  dimension "d194" = 10
  dimension "d195" = 10
  dimension "d1" = 3.5
  constraint coincident A0.centre A2.centre
  constraint midpoint A38 L50.end
  constraint midpoint A40 L51.start
  constraint midpoint A36 L52.end
  constraint parallel L50 L51
  constraint parallel L50 L52
  constraint concentric A100 A101
  constraint tangent L51 A102
  constraint tangent A101 A102
  constraint tangent A101 A103
  constraint tangent L52 A103
  constraint equal A102 A103
  measures "d193" diameter of A100
  measures "d194" diameter of A101
  measures "d195" radius of A102
  measures "d1" diameter of A105
extrude "Extruir4" add sketch "Boceto5" against normal up to surface (3 mm away) contours A36 A37 L18 S18 A38 S19 L19 A39 A40 L51 L52 A101 A102 A103
extrude "Extruir5" cut sketch "Boceto5" against normal up to surface (3 mm away) contours A105
move_body "Desplazar4" bodies 1 to x (1, 0, 0) y (0, 1, 0) z (0, 0, 1) at (-3, -79.882, -45)
move_body "Desplazar5" bodies 1 to x (1, 0, 0) y (0, -0.428935, 0.903335) z (0, -0.903335, -0.428935) at (0, 0, 0)
move_body "Desplazar8" bodies 1 to x (1, 0, 0) y (0, 0.707107, 0.707107) z (0, -0.707107, 0.707107) at (0, 0, 0)
sketch "Boceto8" plane through (0, 0, 0) normal (1, 0, 0) x (0, 1, 0)
  circle A0 centre (0, 0) radius 1.75
  circle A1 centre (-38.7828, -16.9438) radius 1.75
  arc A2 (9.4018, 20.4415) -> (8.3195, 20.9054) centre (0, 0) ccw
  arc A3 (8.0358, 21.5443) -> (8.3195, 20.9054) centre (8.5044, 21.37) ccw
  line L0 (8.0358, 21.5443) -> (8.2095, 22.0112)
  spline S0 degree 5 poles (8.2095, 22.0112) (8.2131, 22.0208) (8.22, 22.0402) (8.2297, 22.0694) (8.2412, 22.1089) (8.2537, 22.1588) (8.2649, 22.2091) (8.2752, 22.2597) (8.2851, 22.3105) (8.2946, 22.3613) (8.3038, 22.4123) (8.3126, 22.4634) (8.3208, 22.5147) (8.3284, 22.5662) (8.3353, 22.6178) (8.3416, 22.6697) (8.3473, 22.7217) (8.3526, 22.7738) (8.3576, 22.826) (8.3621, 22.8783) (8.3663, 22.9307) (8.3701, 22.9832) (8.3735, 23.0358) (8.3764, 23.0885) (8.379, 23.1413) (8.3811, 23.1942) (8.3829, 23.2472) (8.3843, 23.3003) (8.3854, 23.3535) (8.3861, 23.4067) (8.3865, 23.4601) (8.3865, 23.5135) (8.3863, 23.5669) (8.3856, 23.6205) (8.3847, 23.6741) (8.3834, 23.7277) (8.3817, 23.7815) (8.3798, 23.8353) (8.3776, 23.8892) (8.375, 23.9431) (8.3721, 23.9971) (8.369, 24.0511) (8.3655, 24.1052) (8.3617, 24.1593) (8.3576, 24.2135) (8.3533, 24.2678) (8.3486, 24.3221) (8.3437, 24.3764) (8.3384, 24.4308) (8.3329, 24.4852) (8.3271, 24.5397) (8.321, 24.5942) (8.3147, 24.6487) (8.308, 24.7033) (8.3011, 24.758) (8.2939, 24.8126) (8.2865, 24.8673) (8.2787, 24.9221) (8.2707, 24.9768) (8.2625, 25.0316) (8.254, 25.0865) (8.2452, 25.1413) (8.2361, 25.1962) (8.2268, 25.2511) (8.2172, 25.3061) (8.2074, 25.361) (8.1973, 25.416) (8.187, 25.471) (8.1764, 25.5261) (8.1655, 25.5811) (8.1544, 25.6362) (8.1453, 25.6803) (8.1384, 25.7134) (8.1338, 25.7354) (8.1314, 25.7465) knots 0 0 0 0 0 0 0.01428571 0.02857143 0.04285714 0.05714286 0.07142857 0.08571429 0.1 0.11428571 0.12857143 0.14285714 0.15714286 0.17142857 0.18571429 0.2 0.21428571 0.22857143 0.24285714 0.25714286 0.27142857 0.28571429 0.3 0.31428571 0.32857143 0.34285714 0.35714286 0.37142857 0.38571429 0.4 0.41428571 0.42857143 0.44285714 0.45714286 0.47142857 0.48571429 0.5 0.51428571 0.52857143 0.54285714 0.55714286 0.57142857 0.58571429 0.6 0.61428571 0.62857143 0.64285714 0.65714286 0.67142857 0.68571429 0.7 0.71428571 0.72857143 0.74285714 0.75714286 0.77142857 0.78571429 0.8 0.81428571 0.82857143 0.84285714 0.85714286 0.87142857 0.88571429 0.9 0.91428571 0.92857143 0.94285714 0.95714286 0.97142857 0.98571429 1 1 1 1 1 1
  arc A4 (8.1314, 25.7465) -> (6.7477, 26.1432) centre (0, 0) ccw
  spline S1 degree 5 poles (6.7477, 26.1432) (6.7399, 26.1351) (6.7242, 26.1189) (6.7008, 26.0945) (6.6698, 26.0619) (6.6312, 26.0211) (6.5928, 25.9802) (6.5547, 25.9391) (6.5167, 25.8979) (6.479, 25.8566) (6.4416, 25.8152) (6.4043, 25.7737) (6.3673, 25.7321) (6.3306, 25.6903) (6.294, 25.6485) (6.2578, 25.6065) (6.2217, 25.5644) (6.1859, 25.5222) (6.1503, 25.4798) (6.115, 25.4374) (6.08, 25.3949) (6.0452, 25.3522) (6.0106, 25.3094) (5.9763, 25.2665) (5.9423, 25.2235) (5.9085, 25.1804) (5.8749, 25.1372) (5.8417, 25.0938) (5.8087, 25.0504) (5.776, 25.0068) (5.7435, 24.9631) (5.7114, 24.9193) (5.6795, 24.8754) (5.6479, 24.8314) (5.6165, 24.7872) (5.5855, 24.743) (5.5548, 24.6986) (5.5243, 24.6541) (5.4941, 24.6095) (5.4643, 24.5648) (5.4348, 24.5199) (5.4055, 24.475) (5.3766, 24.4299) (5.348, 24.3847) (5.3198, 24.3394) (5.2919, 24.294) (5.2643, 24.2485) (5.237, 24.2028) (5.21, 24.157) (5.1835, 24.1112) (5.1572, 24.0651) (5.1314, 24.019) (5.106, 23.9727) (5.081, 23.9263) (5.0564, 23.8798) (5.0322, 23.8331) (5.0083, 23.7864) (4.9848, 23.7395) (4.9617, 23.6925) (4.939, 23.6453) (4.9169, 23.5981) (4.8954, 23.5506) (4.8745, 23.5029) (4.8543, 23.4551) (4.8347, 23.4071) (4.8155, 23.359) (4.7966, 23.3108) (4.7781, 23.2625) (4.76, 23.2141) (4.7428, 23.1655) (4.727, 23.1166) (4.7159, 23.077) (4.7086, 23.0471) (4.7042, 23.027) (4.7021, 23.0169) knots -1 -1 -1 -1 -1 -1 -0.98571429 -0.97142857 -0.95714286 -0.94285714 -0.92857143 -0.91428571 -0.9 -0.88571429 -0.87142857 -0.85714286 -0.84285714 -0.82857143 -0.81428571 -0.8 -0.78571429 -0.77142857 -0.75714286 -0.74285714 -0.72857143 -0.71428571 -0.7 -0.68571429 -0.67142857 -0.65714286 -0.64285714 -0.62857143 -0.61428571 -0.6 -0.58571429 -0.57142857 -0.55714286 -0.54285714 -0.52857143 -0.51428571 -0.5 -0.48571429 -0.47142857 -0.45714286 -0.44285714 -0.42857143 -0.41428571 -0.4 -0.38571429 -0.37142857 -0.35714286 -0.34285714 -0.32857143 -0.31428571 -0.3 -0.28571429 -0.27142857 -0.25714286 -0.24285714 -0.22857143 -0.21428571 -0.2 -0.18571429 -0.17142857 -0.15714286 -0.14285714 -0.12857143 -0.11428571 -0.1 -0.08571429 -0.07142857 -0.05714286 -0.04285714 -0.02857143 -0.01428571 0 0 0 0 0 0
  line L1 (4.7021, 23.0169) -> (4.602, 22.5289)
  arc A5 (4.0228, 22.1375) -> (4.602, 22.5289) centre (4.1122, 22.6294) ccw
  arc A6 (4.0228, 22.1375) -> (2.8592, 22.3176) centre (0, 0) ccw
  arc A7 (2.4255, 22.8659) -> (2.8592, 22.3176) centre (2.9227, 22.8135) ccw
  line L2 (2.4255, 22.8659) -> (2.4776, 23.3613)
  spline S2 degree 5 poles (2.4776, 23.3613) (2.4787, 23.3715) (2.4806, 23.392) (2.4827, 23.4227) (2.484, 23.4638) (2.4838, 23.5152) (2.4821, 23.5668) (2.4795, 23.6183) (2.4764, 23.67) (2.473, 23.7216) (2.4692, 23.7733) (2.465, 23.825) (2.4602, 23.8767) (2.4548, 23.9284) (2.4486, 23.9802) (2.4418, 24.0319) (2.4345, 24.0837) (2.4266, 24.1355) (2.4184, 24.1873) (2.4098, 24.2391) (2.4008, 24.2909) (2.3914, 24.3427) (2.3816, 24.3945) (2.3714, 24.4463) (2.3607, 24.4981) (2.3497, 24.5499) (2.3382, 24.6016) (2.3264, 24.6534) (2.3142, 24.7052) (2.3016, 24.7569) (2.2887, 24.8087) (2.2755, 24.8604) (2.2619, 24.9121) (2.248, 24.9638) (2.2337, 25.0155) (2.2191, 25.0672) (2.2042, 25.1188) (2.1889, 25.1704) (2.1734, 25.222) (2.1575, 25.2736) (2.1413, 25.3252) (2.1248, 25.3768) (2.108, 25.4283) (2.0908, 25.4798) (2.0734, 25.5313) (2.0557, 25.5827) (2.0377, 25.6342) (2.0194, 25.6856) (2.0008, 25.7369) (1.9819, 25.7883) (1.9627, 25.8396) (1.9433, 25.8909) (1.9236, 25.9421) (1.9035, 25.9934) (1.8833, 26.0445) (1.8627, 26.0957) (1.8419, 26.1468) (1.8208, 26.1979) (1.7994, 26.249) (1.7778, 26.3) (1.7559, 26.351) (1.7337, 26.4019) (1.7113, 26.4529) (1.6886, 26.5037) (1.6657, 26.5546) (1.6425, 26.6054) (1.6191, 26.6561) (1.5954, 26.7068) (1.5714, 26.7575) (1.5472, 26.8081) (1.5228, 26.8587) (1.503, 26.8992) (1.4881, 26.9295) (1.4781, 26.9497) (1.4731, 26.9598) knots 0 0 0 0 0 0 0.01428571 0.02857143 0.04285714 0.05714286 0.07142857 0.08571429 0.1 0.11428571 0.12857143 0.14285714 0.15714286 0.17142857 0.18571429 0.2 0.21428571 0.22857143 0.24285714 0.25714286 0.27142857 0.28571429 0.3 0.31428571 0.32857143 0.34285714 0.35714286 0.37142857 0.38571429 0.4 0.41428571 0.42857143 0.44285714 0.45714286 0.47142857 0.48571429 0.5 0.51428571 0.52857143 0.54285714 0.55714286 0.57142857 0.58571429 0.6 0.61428571 0.62857143 0.64285714 0.65714286 0.67142857 0.68571429 0.7 0.71428571 0.72857143 0.74285714 0.75714286 0.77142857 0.78571429 0.8 0.81428571 0.82857143 0.84285714 0.85714286 0.87142857 0.88571429 0.9 0.91428571 0.92857143 0.94285714 0.95714286 0.97142857 0.98571429 1 1 1 1 1 1
  arc A8 (1.4731, 26.9598) -> (0.0342, 27) centre (0, 0) ccw
  spline S3 degree 5 poles (0.0342, 27) (0.0286, 26.9902) (0.0175, 26.9706) (0.0009, 26.9411) (-0.0211, 26.9019) (-0.0483, 26.8527) (-0.0753, 26.8035) (-0.1021, 26.7543) (-0.1286, 26.7049) (-0.1548, 26.6556) (-0.1808, 26.6061) (-0.2065, 26.5567) (-0.232, 26.5071) (-0.2572, 26.4576) (-0.2822, 26.4079) (-0.3069, 26.3582) (-0.3314, 26.3085) (-0.3555, 26.2587) (-0.3795, 26.2089) (-0.4031, 26.159) (-0.4265, 26.1091) (-0.4496, 26.0591) (-0.4724, 26.0091) (-0.495, 25.959) (-0.5173, 25.9089) (-0.5393, 25.8587) (-0.561, 25.8085) (-0.5824, 25.7582) (-0.6036, 25.7079) (-0.6244, 25.6576) (-0.645, 25.6072) (-0.6653, 25.5568) (-0.6852, 25.5063) (-0.7049, 25.4558) (-0.7242, 25.4053) (-0.7433, 25.3547) (-0.762, 25.304) (-0.7805, 25.2534) (-0.7986, 25.2027) (-0.8164, 25.1519) (-0.8339, 25.1012) (-0.851, 25.0504) (-0.8678, 24.9995) (-0.8842, 24.9486) (-0.9003, 24.8977) (-0.9161, 24.8468) (-0.9315, 24.7958) (-0.9465, 24.7448) (-0.9613, 24.6938) (-0.9756, 24.6427) (-0.9895, 24.5916) (-1.0031, 24.5405) (-1.0162, 24.4894) (-1.0289, 24.4382) (-1.0411, 24.387) (-1.053, 24.3358) (-1.0645, 24.2846) (-1.0756, 24.2333) (-1.0863, 24.1821) (-1.0965, 24.1308) (-1.1062, 24.0795) (-1.1152, 24.0281) (-1.1236, 23.9768) (-1.1312, 23.9254) (-1.1383, 23.874) (-1.1449, 23.8227) (-1.1512, 23.7713) (-1.1572, 23.7199) (-1.1627, 23.6686) (-1.1672, 23.6172) (-1.1704, 23.5659) (-1.1713, 23.5248) (-1.171, 23.494) (-1.1702, 23.4734) (-1.1697, 23.4632) knots -1 -1 -1 -1 -1 -1 -0.98571429 -0.97142857 -0.95714286 -0.94285714 -0.92857143 -0.91428571 -0.9 -0.88571429 -0.87142857 -0.85714286 -0.84285714 -0.82857143 -0.81428571 -0.8 -0.78571429 -0.77142857 -0.75714286 -0.74285714 -0.72857143 -0.71428571 -0.7 -0.68571429 -0.67142857 -0.65714286 -0.64285714 -0.62857143 -0.61428571 -0.6 -0.58571429 -0.57142857 -0.55714286 -0.54285714 -0.52857143 -0.51428571 -0.5 -0.48571429 -0.47142857 -0.45714286 -0.44285714 -0.42857143 -0.41428571 -0.4 -0.38571429 -0.37142857 -0.35714286 -0.34285714 -0.32857143 -0.31428571 -0.3 -0.28571429 -0.27142857 -0.25714286 -0.24285714 -0.22857143 -0.21428571 -0.2 -0.18571429 -0.17142857 -0.15714286 -0.14285714 -0.12857143 -0.11428571 -0.1 -0.08571429 -0.07142857 -0.05714286 -0.04285714 -0.02857143 -0.01428571 0 0 0 0 0 0
  line L3 (-1.1697, 23.4632) -> (-1.1453, 22.9656)
  arc A9 (-1.6089, 22.4424) -> (-1.1453, 22.9656) centre (-1.6447, 22.9411) ccw
  arc A10 (-1.6089, 22.4424) -> (-2.7808, 22.3275) centre (0, 0) ccw
  arc A11 (-3.3373, 22.7507) -> (-2.7808, 22.3275) centre (-2.8426, 22.8237) ccw
  line L4 (-3.3373, 22.7507) -> (-3.4099, 23.2435)
  spline S4 degree 5 poles (-3.4099, 23.2435) (-3.4114, 23.2537) (-3.4147, 23.274) (-3.4203, 23.3043) (-3.4292, 23.3444) (-3.4423, 23.3942) (-3.4567, 23.4436) (-3.4721, 23.493) (-3.4879, 23.5422) (-3.504, 23.5914) (-3.5205, 23.6405) (-3.5374, 23.6895) (-3.5549, 23.7384) (-3.5731, 23.7871) (-3.5919, 23.8357) (-3.6114, 23.8842) (-3.6314, 23.9325) (-3.6519, 23.9807) (-3.6727, 24.0288) (-3.6939, 24.0769) (-3.7155, 24.1248) (-3.7375, 24.1726) (-3.7599, 24.2204) (-3.7827, 24.268) (-3.8059, 24.3155) (-3.8295, 24.3629) (-3.8534, 24.4102) (-3.8778, 24.4574) (-3.9025, 24.5045) (-3.9275, 24.5515) (-3.9528, 24.5984) (-3.9785, 24.6452) (-4.0045, 24.692) (-4.0309, 24.7386) (-4.0575, 24.7851) (-4.0845, 24.8315) (-4.1118, 24.8778) (-4.1395, 24.924) (-4.1674, 24.9701) (-4.1956, 25.0162) (-4.2241, 25.0621) (-4.2529, 25.1079) (-4.282, 25.1536) (-4.3114, 25.1993) (-4.3411, 25.2448) (-4.3711, 25.2902) (-4.4013, 25.3356) (-4.4318, 25.3808) (-4.4626, 25.4259) (-4.4936, 25.471) (-4.525, 25.5159) (-4.5566, 25.5607) (-4.5884, 25.6055) (-4.6205, 25.6501) (-4.6529, 25.6947) (-4.6855, 25.7391) (-4.7184, 25.7834) (-4.7516, 25.8277) (-4.785, 25.8718) (-4.8186, 25.9159) (-4.8525, 25.9598) (-4.8866, 26.0036) (-4.921, 26.0474) (-4.9556, 26.091) (-4.9905, 26.1346) (-5.0256, 26.178) (-5.0609, 26.2213) (-5.0965, 26.2645) (-5.1323, 26.3077) (-5.1683, 26.3507) (-5.2046, 26.3936) (-5.2338, 26.4279) (-5.2558, 26.4535) (-5.2705, 26.4706) (-5.2778, 26.4791) knots 0 0 0 0 0 0 0.01428571 0.02857143 0.04285714 0.05714286 0.07142857 0.08571429 0.1 0.11428571 0.12857143 0.14285714 0.15714286 0.17142857 0.18571429 0.2 0.21428571 0.22857143 0.24285714 0.25714286 0.27142857 0.28571429 0.3 0.31428571 0.32857143 0.34285714 0.35714286 0.37142857 0.38571429 0.4 0.41428571 0.42857143 0.44285714 0.45714286 0.47142857 0.48571429 0.5 0.51428571 0.52857143 0.54285714 0.55714286 0.57142857 0.58571429 0.6 0.61428571 0.62857143 0.64285714 0.65714286 0.67142857 0.68571429 0.7 0.71428571 0.72857143 0.74285714 0.75714286 0.77142857 0.78571429 0.8 0.81428571 0.82857143 0.84285714 0.85714286 0.87142857 0.88571429 0.9 0.91428571 0.92857143 0.94285714 0.95714286 0.97142857 0.98571429 1 1 1 1 1 1
  arc A12 (-5.2778, 26.4791) -> (-6.6815, 26.1602) centre (0, 0) ccw
  spline S5 degree 5 poles (-6.6815, 26.1602) (-6.6845, 26.1493) (-6.6904, 26.1276) (-6.6991, 26.095) (-6.7107, 26.0514) (-6.7248, 25.9971) (-6.7387, 25.9427) (-6.7524, 25.8883) (-6.7658, 25.834) (-6.7789, 25.7796) (-6.7918, 25.7253) (-6.8044, 25.671) (-6.8168, 25.6167) (-6.8289, 25.5624) (-6.8407, 25.5081) (-6.8523, 25.4538) (-6.8636, 25.3996) (-6.8746, 25.3453) (-6.8854, 25.2911) (-6.8959, 25.2369) (-6.9061, 25.1827) (-6.9161, 25.1286) (-6.9258, 25.0744) (-6.9352, 25.0203) (-6.9443, 24.9662) (-6.9531, 24.9122) (-6.9617, 24.8581) (-6.9699, 24.8041) (-6.9779, 24.7502) (-6.9856, 24.6962) (-6.993, 24.6423) (-7.0001, 24.5884) (-7.0069, 24.5346) (-7.0133, 24.4808) (-7.0195, 24.427) (-7.0254, 24.3733) (-7.031, 24.3196) (-7.0362, 24.2659) (-7.0412, 24.2123) (-7.0458, 24.1587) (-7.0501, 24.1052) (-7.054, 24.0517) (-7.0576, 23.9983) (-7.0609, 23.9449) (-7.0638, 23.8916) (-7.0664, 23.8384) (-7.0687, 23.7852) (-7.0706, 23.732) (-7.0722, 23.6789) (-7.0733, 23.6259) (-7.0741, 23.573) (-7.0745, 23.5201) (-7.0745, 23.4673) (-7.0741, 23.4146) (-7.0732, 23.362) (-7.072, 23.3094) (-7.0703, 23.2569) (-7.0684, 23.2045) (-7.066, 23.1522) (-7.0631, 23.1) (-7.0598, 23.0479) (-7.0557, 22.9959) (-7.0511, 22.9441) (-7.0457, 22.8924) (-7.0398, 22.8409) (-7.0334, 22.7895) (-7.0268, 22.7382) (-7.0197, 22.6869) (-7.0123, 22.6358) (-7.0039, 22.585) (-6.9942, 22.5344) (-6.9849, 22.4944) (-6.9769, 22.4647) (-6.971, 22.445) (-6.968, 22.4351) knots -1 -1 -1 -1 -1 -1 -0.98571429 -0.97142857 -0.95714286 -0.94285714 -0.92857143 -0.91428571 -0.9 -0.88571429 -0.87142857 -0.85714286 -0.84285714 -0.82857143 -0.81428571 -0.8 -0.78571429 -0.77142857 -0.75714286 -0.74285714 -0.72857143 -0.71428571 -0.7 -0.68571429 -0.67142857 -0.65714286 -0.64285714 -0.62857143 -0.61428571 -0.6 -0.58571429 -0.57142857 -0.55714286 -0.54285714 -0.52857143 -0.51428571 -0.5 -0.48571429 -0.47142857 -0.45714286 -0.44285714 -0.42857143 -0.41428571 -0.4 -0.38571429 -0.37142857 -0.35714286 -0.34285714 -0.32857143 -0.31428571 -0.3 -0.28571429 -0.27142857 -0.25714286 -0.24285714 -0.22857143 -0.21428571 -0.2 -0.18571429 -0.17142857 -0.15714286 -0.14285714 -0.12857143 -0.11428571 -0.1 -0.08571429 -0.07142857 -0.05714286 -0.04285714 -0.02857143 -0.01428571 0 0 0 0 0 0
  line L5 (-6.968, 22.4351) -> (-6.8206, 21.9593)
  arc A13 (-7.1396, 21.3372) -> (-6.8206, 21.9593) centre (-7.2982, 21.8114) ccw
  arc A14 (-7.1396, 21.3372) -> (-8.2461, 20.9345) centre (0, 0) ccw
  arc A15 (-8.8903, 21.206) -> (-8.2461, 20.9345) centre (-8.4293, 21.3997) ccw
  line L6 (-8.8903, 21.206) -> (-9.0832, 21.6653)
  spline S6 degree 5 poles (-9.0832, 21.6653) (-9.0872, 21.6747) (-9.0954, 21.6936) (-9.1084, 21.7215) (-9.127, 21.7582) (-9.152, 21.8031) (-9.1783, 21.8475) (-9.2054, 21.8914) (-9.233, 21.9352) (-9.2609, 21.9788) (-9.2891, 22.0222) (-9.3176, 22.0655) (-9.3467, 22.1085) (-9.3765, 22.1512) (-9.4068, 22.1936) (-9.4377, 22.2357) (-9.4691, 22.2775) (-9.5009, 22.3191) (-9.5331, 22.3606) (-9.5656, 22.4018) (-9.5984, 22.4429) (-9.6316, 22.4837) (-9.6651, 22.5244) (-9.699, 22.5649) (-9.7333, 22.6051) (-9.768, 22.6452) (-9.8029, 22.685) (-9.8383, 22.7247) (-9.8739, 22.7642) (-9.9098, 22.8035) (-9.946, 22.8426) (-9.9825, 22.8816) (-10.0194, 22.9203) (-10.0565, 22.9589) (-10.0939, 22.9973) (-10.1316, 23.0356) (-10.1695, 23.0737) (-10.2078, 23.1116) (-10.2463, 23.1493) (-10.2851, 23.1868) (-10.3241, 23.2242) (-10.3634, 23.2614) (-10.403, 23.2985) (-10.4428, 23.3354) (-10.4828, 23.3721) (-10.5232, 23.4086) (-10.5637, 23.445) (-10.6045, 23.4813) (-10.6456, 23.5173) (-10.6868, 23.5532) (-10.7284, 23.589) (-10.7701, 23.6245) (-10.8121, 23.6599) (-10.8543, 23.6952) (-10.8967, 23.7303) (-10.9394, 23.7652) (-10.9823, 23.8) (-11.0254, 23.8346) (-11.0687, 23.869) (-11.1122, 23.9033) (-11.156, 23.9375) (-11.1999, 23.9714) (-11.2441, 24.0052) (-11.2885, 24.0389) (-11.3331, 24.0724) (-11.3779, 24.1057) (-11.4229, 24.1389) (-11.4681, 24.172) (-11.5135, 24.2048) (-11.5591, 24.2375) (-11.6049, 24.2701) (-11.6417, 24.296) (-11.6694, 24.3154) (-11.6879, 24.3283) (-11.6971, 24.3347) knots 0 0 0 0 0 0 0.01428571 0.02857143 0.04285714 0.05714286 0.07142857 0.08571429 0.1 0.11428571 0.12857143 0.14285714 0.15714286 0.17142857 0.18571429 0.2 0.21428571 0.22857143 0.24285714 0.25714286 0.27142857 0.28571429 0.3 0.31428571 0.32857143 0.34285714 0.35714286 0.37142857 0.38571429 0.4 0.41428571 0.42857143 0.44285714 0.45714286 0.47142857 0.48571429 0.5 0.51428571 0.52857143 0.54285714 0.55714286 0.57142857 0.58571429 0.6 0.61428571 0.62857143 0.64285714 0.65714286 0.67142857 0.68571429 0.7 0.71428571 0.72857143 0.74285714 0.75714286 0.77142857 0.78571429 0.8 0.81428571 0.82857143 0.84285714 0.85714286 0.87142857 0.88571429 0.9 0.91428571 0.92857143 0.94285714 0.95714286 0.97142857 0.98571429 1 1 1 1 1 1
  arc A16 (-11.6971, 24.3347) -> (-12.9774, 23.6767) centre (0, 0) ccw